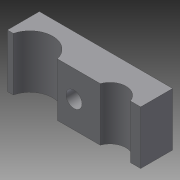
# Autodesk Inventor part: Крепление кабеля
Saved by Autodesk Inventor 2014 (Build 180170000, 170)
## iProperties
Created: 2017-03-03
Part Number: Крепление кабеля
Material: Типовые
Document SubType Name: Modeling
Designer: Nikopol
Density: 1 g/cm^3
Appearance: По умолчанию
Author: Nikopol
Autodesk Inventor part; units mm, degrees
ref_plane "YZ Plane" through (0, 0, 0) normal (1, 0, 0) x (0, 1, 0)
ref_plane "XZ Plane" through (0, 0, 0) normal (0, 1, 0) x (-1, 0, 0)
ref_plane "XY Plane" through (0, 0, 0) normal (0, 0, 1) x (1, 0, 0)
sketch "Эскиз1" plane through (0, 0, 0) normal (0, 0, 1) x (1, 0, 0)
  line L0 (-12.5, 3) -> (12.5, 3)
  line L1 (12.5, 3) -> (12.5, -3)
  line L2 (-12.5, -3) -> (-12.5, 3)
  arc A0 (10.5784, -3) -> (4.9216, -3) centre (7.75, -4) ccw
  arc A1 (-3.1193, -3) -> (-11.3807, -3) centre (-7.25, -4) ccw
  line L3 (12.5, -3) -> (10.5784, -3)
  line L4 (4.9216, -3) -> (-3.1193, -3)
  line L5 (-11.3807, -3) -> (-12.5, -3)
  point P0 (0, 0)
  point P1 (-12.5, 0)
  point P2 (0, 3)
  dimension "d0" = 25
  dimension "d1" = 6
  dimension "d2" = 6
  dimension "d3" = 8.5
  dimension "d7" = 5.25
  dimension "d8" = 15
  constraints: 12 end point, 4 parallel, 4 point on circle, 2 centre point, 2 midpoint, 1 horizontal, 1 horizontal alignment, 1 perpendicular, 1 vertical alignment
  measures "d0" distance of L1.end L2.start
  measures "d1" distance of L0.end L1.end
  measures "d2" diameter of A0
  measures "d3" diameter of A1
  measures "d7" distance from line of L2 A1.centre
  measures "d8" distance of A0.centre A1.centre
extrude "Выдавливание1" add sketch "Эскиз1" along normal blind 10
sketch "Эскиз2" plane through (-12.5, 3, 0) normal (0, 1, 0) x (1, 0, 0)
  point P0 (12.5, 0)
  point P1 (12.5, -5)
hole "Отверстие1" at (0, 3, 5) direction (0, -1, 0) diameter 3 end through all
